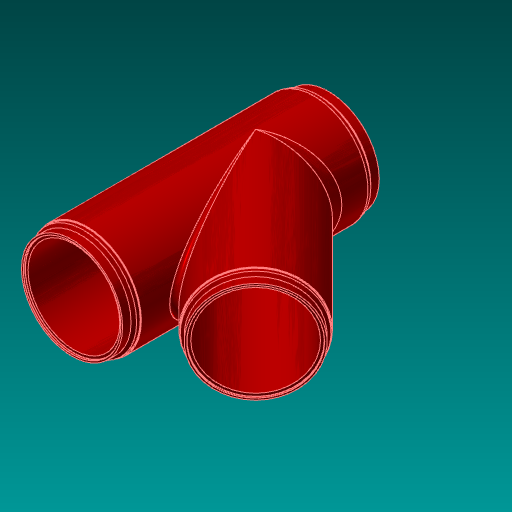
# Autodesk Inventor part: A1-19037-300-05 HCWI lateral
Saved by Autodesk Inventor 2017.3 (Build 213256000, 256)
## iProperties
Created: 2019-08-22
Part Number: A1-19037-300-05 HCWI lateral
Material: Iron, HCWI
Document SubType Name: Modeling
Designer: GVD
Density: 7.33517 g/cm^3
Appearance: Iron Gray(1)
Project: A1-19037--CNUL Albian CST laterals
Mass: 2.01918e+06 g
Surface Area: 103208 cm^2
Volume: 275273 cm^3
Constructed By: Graeme_Van_Dongen
Project Name: CST laterals
Author: GVD
Autodesk Inventor part; units mm, degrees
ref_plane "YZ Plane" through (0, 0, 0) normal (1, 0, 0) x (0, 1, 0)
ref_plane "XZ Plane" through (0, 0, 0) normal (0, 1, 0) x (-1, 0, 0)
sketch "Sketch1" plane through (0, 0, 0) normal (0, 0, 1) x (1, 0, 0)
  circle A0 centre (0, 0) radius 311.15
  circle A1 centre (0, 0) radius 342.9
  circle A2 centre (0, 0) radius 368.3
  dimension "d0" = 622.3
  dimension "d1" = 685.8
  dimension "d2" = 736.6
  constraints: 3 centre point, 3 coincident
  measures "d0" diameter of A0
  measures "d1" diameter of A1
  measures "d2" diameter of A2
extrude "Extrusion1" add sketch "Sketch1" along normal blind 1245.2 and the other way blind 495.2 contours A0 | A1
ref_plane "Work Plane1" through (0, 0, 0) normal (0.7071068, 0, 0.7071068) x (0, 1, 0)
sketch "Sketch2" plane through (0, 0, 0) normal (0.7071068, 0, 0.7071068) x (0, 1, 0)
  circle A0 centre (0, 0) radius 311.15
  circle A1 centre (0, 0) radius 342.9
  circle A2 centre (0, 0) radius 368.3
  dimension "d8" = 622.3
  dimension "d9" = 685.8
  dimension "d10" = 736.6
  constraints: 3 centre point, 3 coincident
  measures "d8" diameter of A0
  measures "d9" diameter of A1
  measures "d10" diameter of A2
extrude "Extrusion2" add sketch "Sketch2" along normal blind 1245.2 contours A0 | A1
sketch "Sketch3" plane through (0, 0, -495.2) normal (0, 0, -1) x (-1, 0, 0)
  circle A0 centre (0, 0) radius 330.2
  dimension "d13" = 660.4
  constraints: 1 centre point, 1 coincident
  measures "d13" diameter of A0
extrude "Extrusion3" cut sketch "Sketch3" against normal blind 12.7
sketch "Sketch4" plane through (0, 0, 1245.2) normal (0, 0, 1) x (1, 0, 0)
  circle A0 centre (0, 0) radius 330.2
  dimension "d16" = 660.4
  constraints: 1 centre point, 1 coincident
  measures "d16" diameter of A0
extrude "Extrusion4" cut sketch "Sketch4" against normal blind 12.7
sketch "Sketch5" plane through (880.4894, 0, 880.4894) normal (0.7071068, 0, 0.7071068) x (0.7071068, 0, -0.7071068)
  circle A0 centre (0, 0) radius 330.2
  point P0 (0, 0)
  dimension "d19" = 660.4
  constraints: 1 centre point, 1 coincident
  measures "d19" diameter of A0
extrude "Extrusion5" cut sketch "Sketch5" against normal blind 12.7
extrude "Extrusion6" add sketch "Sketch1" along normal blind 1169 and the other way blind 419 contours A2
extrude "Extrusion7" add sketch "Sketch2" along normal blind 1169 contours A2
extrude "Extrusion8" cut sketch "Sketch1" along normal through all both and the other way through all contours A0
extrude "Extrusion9" cut sketch "Sketch2" along normal through all contours A0
fillet "Fillet1" radius 25.4 2 edges at (260.4274, 260.4274, 628.7274) (260.4274, -260.4274, 628.7274)
fillet "Fillet2" radius 152.4 2 edges at (260.4274, -260.4274, -107.8726) (260.4274, 260.4274, -107.8726)
fillet "Fillet3" radius 25.4 2 edges at (220.0163, 220.0163, 531.1663) (220.0163, -220.0163, 531.1663)
fillet "Fillet4" radius 25.4 2 edges at (220.0163, -220.0163, -91.1337) (220.0163, 220.0163, -91.1337)
sketch "Sketch6" plane through (0, 0, 1169) normal (0, 0, 1) x (1, 0, 0)
  circle A0 centre (0, 0) radius 368.3 projected
  circle A1 centre (0, 0) radius 361.696
  dimension "d39" = 723.392
  constraints: 1 centre point, 1 coincident
  measures "d39" diameter of A1
extrude "Extrusion10" cut sketch "Sketch6" against normal blind 25.4
sketch "Sketch7" plane through (0, 0, -419) normal (0, 0, -1) x (-1, 0, 0)
  circle A0 centre (0, 0) radius 368.3 projected
  circle A1 centre (0, 0) radius 361.696
  dimension "d42" = 723.392
  constraints: 1 centre point, 1 coincident
  measures "d42" diameter of A1
extrude "Extrusion11" cut sketch "Sketch7" against normal blind 25.4
sketch "Sketch8" plane through (826.6078, 0, 826.6078) normal (0.7071068, 0, 0.7071068) x (0.7071068, 0, -0.7071068)
  circle A0 centre (0, 0) radius 368.3 projected
  circle A1 centre (0, 0) radius 361.696
  point P0 (0, 0)
  dimension "d45" = 723.392
  constraints: 1 centre point, 1 coincident
  measures "d45" diameter of A1
extrude "Extrusion12" cut sketch "Sketch8" against normal blind 25.4
fillet "Fillet5" radius 0.7937 3 edges at (552.8882, 0, 1064.4036) (-361.696, 0, 1143.6) (361.696, 0, -393.6)
chamfer "Chamfer2" distance 18.796 angle 45 3 edges at (-342.9, 0, 1169) (826.6078, -342.9, 826.6078) (-342.9, 0, -419)
fillet "Fillet6" radius 0.7937 3 edges at (-330.2, 0, 1232.5) (638.021, 0, 1104.9944) (330.2, 0, -482.5)
chamfer "Chamfer3" distance 0.7937 angle 45 3 edges at (330.2, 0, -495.2) (-330.2, 0, 1245.2) (647.0027, 0, 1113.976)
equation "\"d8\" = d0"
equation "\"d9\" = d1"
equation "\"d10\" = d2"
equation "\"d16\" = d13"
equation "\"d17\" = d14"
equation "\"d19\" = d13"
equation "\"d20\" = d14"
equation "\"d28\" = d11"
equation "\"d30\" = d11"
equation "\"d42\" = d39"
equation "\"d45\" = d39"
equation "\"d49\" = -0.5 * d1 + 0.5 * d39"
equation "\"d14\" = 12.7"
equation "\"d11\" = 1245.2"
body "Solid1"
